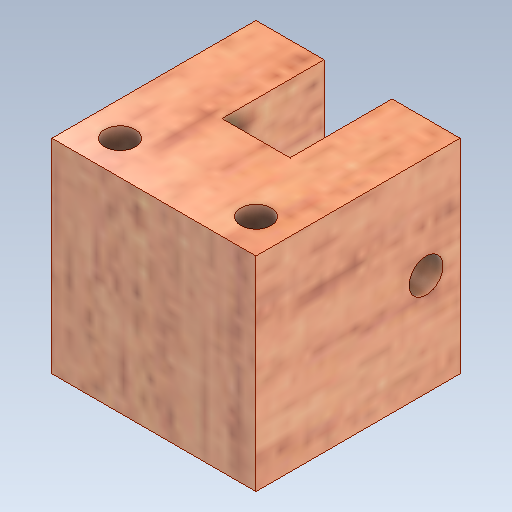
# Autodesk Inventor part: 0005-10-019 intinzator y
Saved by Autodesk Inventor 2020 (Build 240168000, 168)
## iProperties
Created: 2020-12-19
Part Number: 0005-10-019 intinzator y
Material: Generic
Document SubType Name: Modeling
Designer: Iulian Bors
Density: 1 g/cm^3
Appearance: Red Oak - Natural Low Gloss
Author: Iulian Bors
Subject: 019
Autodesk Inventor part; units mm, degrees
ref_plane "YZ Plane" through (0, 0, 0) normal (1, 0, 0) x (0, 1, 0)
ref_plane "XZ Plane" through (0, 0, 0) normal (0, 1, 0) x (-1, 0, 0)
ref_plane "XY Plane" through (0, 0, 0) normal (0, 0, 1) x (1, 0, 0)
sketch "Sketch1" plane through (0, 0, 0) normal (0, 0, 1) x (1, 0, 0)
  line L0 (-15, 15) -> (15, 15)
  line L1 (15, 15) -> (15, -15)
  line L2 (15, -15) -> (-15, -15)
  line L3 (-15, -15) -> (-15, 15)
  point P0 (0, 0)
  point P1 (0, 15)
  point P2 (-15, 0)
  dimension "d0" = 30
  dimension "d1" = 30
  constraints: 8 end point, 2 midpoint, 2 parallel, 1 horizontal, 1 horizontal alignment, 1 perpendicular, 1 vertical alignment
  measures "d0" distance of L0.start L0.end
  measures "d1" distance of L0.end L1.end
extrude "Extrusion1" add sketch "Sketch1" along normal blind 30
sketch "Sketch4" plane through (0, 0, 0) normal (0, 0, -1) x (-1, 0, 0)
  line L0 (5, -15) -> (-5, -15)
  line L1 (-5, -15) -> (-5, 15)
  line L2 (-5, 15) -> (5, 15)
  line L3 (5, 15) -> (5, -15)
  line L4 (15, -15) -> (-15, -15) projected
  line L5 (-15, 15) -> (15, 15) projected
  point P0 (0, 0)
  point P1 (0, -15)
  dimension "d8" = 10
  constraints: 8 end point, 2 collinear, 2 parallel, 1 horizontal, 1 midpoint, 1 perpendicular, 1 vertical alignment
  measures "d8" distance of L0.start L0.end
extrude "Extrusion3" cut sketch "Sketch4" against normal blind 15
sketch "Sketch5" plane through (15, -15, 0) normal (1, 0, 0) x (0, 0, -1)
  line L0 (0, 0) -> (0, 30) projected
  point P0 (0, 15)
  point P1 (-5, 15)
  point P2 (0, 15)
  dimension "d11" = 5
  constraints: 1 horizontal alignment, 1 midpoint
  measures "d11" distance of point (0, 15) point (-5, 15)
hole "Hole1" at (15, 0, 5) direction (-1, 0, 0) diameter 5 end through all
sketch "Sketch8" plane through (15, 15, 30) normal (0, 1, 0) x (1, 0, 0)
  line L0 (0, 0) -> (-30, 0) projected
  line L1 (0, 30) -> (0, 0) projected
  line L2 (0, 30) -> (-10, 30) projected
  line L3 (-10, 30) -> (-10, 15) projected
  line L4 (-10, 15) -> (-20, 15) projected
  line L5 (-20, 15) -> (-20, 30) projected
  line L6 (-20, 30) -> (-30, 30) projected
  circle A0 centre (-25, 5) radius 2.25
  circle A1 centre (-5, 5) radius 2.25
  line L7 (-30, 30) -> (-30, 0) projected
  point P0 (-15, 30)
  dimension "d28" = 4.5
  dimension "d30" = 5
  dimension "d31" = 5
  dimension "d32" = 5
  constraints: 2 centre point, 1 equal radius, 1 horizontal alignment
  measures "d28" diameter of A0
  measures "d30" distance from line of A1.centre L1
  measures "d31" distance from line of A0.centre L7
  measures "d32" distance from line of A0.centre L0
extrude "Extrusion6" cut sketch "Sketch8" against normal through all contours A0 | A1
body "Solid1"
